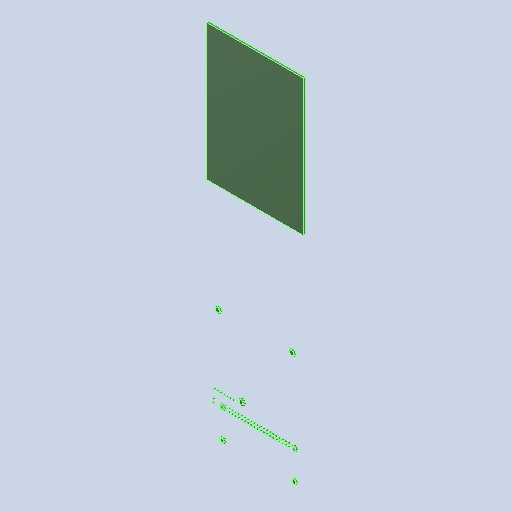
# Autodesk Inventor part: KiCad-OBC.kicad_pcb_Outline
Saved by Autodesk Inventor 2022 (Build 260153000, 153)
## iProperties
Created: 2022-02-26
Part Number: KiCad-OBC.kicad_pcb_Outline
Material: Generic
Document SubType Name: Modeling
Designer: admin
Density: 1 g/cm^3
Appearance: Board Outline
Author: admin
Autodesk Inventor part; units mm, degrees
ref_plane "YZ Plane" through (0, 0, 0) normal (1, 0, 0) x (0, 1, 0)
ref_plane "XZ Plane" through (0, 0, 0) normal (0, 1, 0) x (-1, 0, 0)
ref_plane "XY Plane" through (0, 0, 0) normal (0, 0, 1) x (1, 0, 0)
sketch "Sketch1" plane through (0, 0, 0) normal (0, 0, 1) x (1, 0, 0)
  line L0 (100.6, 36.65) -> (178.3, 36.65)
  line L1 (178.3, 36.65) -> (178.3, 146.7)
  line L2 (178.3, 146.7) -> (100.6, 146.7)
  line L3 (100.6, 146.7) -> (100.6, 36.65)
  circle A0 centre (117.67, -117.87) radius 0.5
  circle A1 centre (117.67, -115.33) radius 0.5
  circle A2 centre (120.21, -117.87) radius 0.5
  circle A3 centre (120.21, -115.33) radius 0.5
  circle A4 centre (122.75, -117.87) radius 0.5
  circle A5 centre (122.75, -115.33) radius 0.5
  circle A6 centre (125.29, -117.87) radius 0.5
  circle A7 centre (125.29, -115.33) radius 0.5
  circle A8 centre (127.83, -117.87) radius 0.5
  circle A9 centre (127.83, -115.33) radius 0.5
  circle A10 centre (130.37, -117.87) radius 0.5
  circle A11 centre (130.37, -115.33) radius 0.5
  circle A12 centre (132.91, -117.87) radius 0.5
  circle A13 centre (132.91, -115.33) radius 0.5
  circle A14 centre (135.45, -117.87) radius 0.5
  circle A15 centre (135.45, -115.33) radius 0.5
  circle A16 centre (137.99, -117.87) radius 0.5
  circle A17 centre (137.99, -115.33) radius 0.5
  circle A18 centre (140.53, -117.87) radius 0.5
  circle A19 centre (140.53, -115.33) radius 0.5
  circle A20 centre (143.07, -117.87) radius 0.5
  circle A21 centre (143.07, -115.33) radius 0.5
  circle A22 centre (145.61, -117.87) radius 0.5
  circle A23 centre (145.61, -115.33) radius 0.5
  circle A24 centre (148.15, -117.87) radius 0.5
  circle A25 centre (148.15, -115.33) radius 0.5
  circle A26 centre (150.69, -117.87) radius 0.5
  circle A27 centre (150.69, -115.33) radius 0.5
  circle A28 centre (153.23, -117.87) radius 0.5
  circle A29 centre (153.23, -115.33) radius 0.5
  circle A30 centre (155.77, -117.87) radius 0.5
  circle A31 centre (155.77, -115.33) radius 0.5
  circle A32 centre (158.31, -117.87) radius 0.5
  circle A33 centre (158.31, -115.33) radius 0.5
  circle A34 centre (160.85, -117.87) radius 0.5
  circle A35 centre (160.85, -115.33) radius 0.5
  circle A36 centre (163.39, -117.87) radius 0.5
  circle A37 centre (163.39, -115.33) radius 0.5
  circle A38 centre (165.93, -117.87) radius 0.5
  circle A39 centre (165.93, -115.33) radius 0.5
  circle A40 centre (166.55, -50.4) radius 0.25
  circle A41 centre (167.2529, -48.7029) radius 0.25
  circle A42 centre (171.35, -50.4) radius 0.25
  circle A43 centre (168.95, -48) radius 0.25
  circle A44 centre (168.95, -52.8) radius 0.25
  circle A45 centre (167.2529, -52.0971) radius 0.25
  circle A46 centre (170.6471, -52.0971) radius 0.25
  circle A47 centre (168.95, -50.4) radius 1.6
  circle A48 centre (170.6471, -48.7029) radius 0.25
  circle A49 centre (106.85, -50.3) radius 0.25
  circle A50 centre (109.25, -50.3) radius 1.6
  circle A51 centre (107.5529, -51.9971) radius 0.25
  circle A52 centre (110.9471, -48.6029) radius 0.25
  circle A53 centre (109.25, -52.7) radius 0.25
  circle A54 centre (111.65, -50.3) radius 0.25
  circle A55 centre (107.5529, -48.6029) radius 0.25
  circle A56 centre (109.25, -47.9) radius 0.25
  circle A57 centre (110.9471, -51.9971) radius 0.25
  circle A58 centre (126.4029, -103.6529) radius 0.25
  circle A59 centre (128.1, -105.35) radius 1.6
  circle A60 centre (129.7971, -107.0471) radius 0.25
  circle A61 centre (128.1, -107.75) radius 0.25
  circle A62 centre (129.7971, -103.6529) radius 0.25
  circle A63 centre (126.4029, -107.0471) radius 0.25
  circle A64 centre (130.5, -105.35) radius 0.25
  circle A65 centre (128.1, -102.95) radius 0.25
  circle A66 centre (125.7, -105.35) radius 0.25
  circle A67 centre (114.825, -116.6) radius 0.25
  circle A68 centre (114.2319, -115.1681) radius 0.25
  circle A69 centre (112.8, -114.575) radius 0.25
  circle A70 centre (111.3681, -118.0319) radius 0.25
  circle A71 centre (112.8, -116.6) radius 1.35
  circle A72 centre (111.3681, -115.1681) radius 0.25
  circle A73 centre (114.2319, -118.0319) radius 0.25
  circle A74 centre (110.775, -116.6) radius 0.25
  circle A75 centre (112.8, -118.625) radius 0.25
  circle A76 centre (169.4181, -138.1181) radius 0.25
  circle A77 centre (168.825, -139.55) radius 0.25
  circle A78 centre (170.85, -137.525) radius 0.25
  circle A79 centre (170.85, -141.575) radius 0.25
  circle A80 centre (169.4181, -140.9819) radius 0.25
  circle A81 centre (172.2819, -140.9819) radius 0.25
  circle A82 centre (172.875, -139.55) radius 0.25
  circle A83 centre (172.2819, -138.1181) radius 0.25
  circle A84 centre (170.85, -139.55) radius 1.35
  circle A85 centre (172.2319, -118.0319) radius 0.25
  circle A86 centre (169.3681, -115.1681) radius 0.25
  circle A87 centre (170.8, -114.575) radius 0.25
  circle A88 centre (168.775, -116.6) radius 0.25
  circle A89 centre (169.3681, -118.0319) radius 0.25
  circle A90 centre (170.8, -116.6) radius 1.35
  circle A91 centre (172.825, -116.6) radius 0.25
  circle A92 centre (170.8, -118.625) radius 0.25
  circle A93 centre (172.2319, -115.1681) radius 0.25
  circle A94 centre (112.8, -139.65) radius 1.35
  circle A95 centre (112.8, -141.675) radius 0.25
  circle A96 centre (114.825, -139.65) radius 0.25
  circle A97 centre (110.775, -139.65) radius 0.25
  circle A98 centre (114.2319, -138.2181) radius 0.25
  circle A99 centre (111.3681, -141.0819) radius 0.25
  circle A100 centre (112.8, -137.625) radius 0.25
  circle A101 centre (111.3681, -138.2181) radius 0.25
  circle A102 centre (114.2319, -141.0819) radius 0.25
  circle A103 centre (105.1, -117.2) radius 0.5
  circle A104 centre (105.1, -114.66) radius 0.5
  circle A105 centre (106.08, -107.32) radius 0.381
  circle A106 centre (108.62, -107.32) radius 0.381
  circle A107 centre (111.16, -107.32) radius 0.381
  circle A108 centre (113.7, -107.32) radius 0.381
  circle A109 centre (116.24, -107.32) radius 0.381
  circle A110 centre (118.78, -107.32) radius 0.381
  circle A111 centre (121.32, -107.32) radius 0.381
  circle A112 centre (112.8, -139.6) radius 1.375
  circle A113 centre (112.8, -116.6) radius 1.375
  circle A114 centre (170.8, -116.6) radius 1.375
  circle A115 centre (170.8, -139.6) radius 1.375
  circle A116 centre (109.1, -50.3) radius 1.6
  circle A117 centre (169.1, -50.3) radius 1.6
  circle A118 centre (128.1, -105.3) radius 1.6
  constraints: 119 centre point, 8 end point
extrude "KiCad-OBC.kicad_pcb_Outline" add sketch "Sketch1" along normal blind 1.6
body "Solid1"
